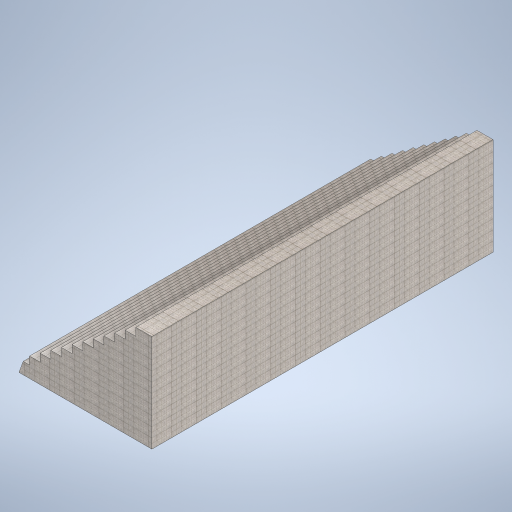
# Autodesk Inventor part: front_stair
Saved by Autodesk Inventor 2024.2 (Build 282272000, 272)
## iProperties
Created: 2024-05-25
Part Number: front_stair
Material: Generic
Document SubType Name: Modeling
Designer: LOSTER_1
Density: 1 g/cm^3
Appearance: Default
Author: LOSTER_1
Autodesk Inventor part; units mm, degrees
ref_plane "YZ Plane" through (0, 0, 0) normal (1, 0, 0) x (0, 1, 0)
ref_plane "XZ Plane" through (0, 0, 0) normal (0, 1, 0) x (-1, 0, 0)
ref_plane "XY Plane" through (0, 0, 0) normal (0, 0, 1) x (1, 0, 0)
sketch "Sketch1" plane through (0, 0, 0) normal (0, 1, 0) x (-1, 0, 0)
  line L0 (1000, 3500) -> (-1000, 3500)
  line L1 (-1000, 3500) -> (-1000, -3500)
  line L2 (-1000, -3500) -> (1000, -3500)
  line L3 (1000, -3500) -> (1000, 3500)
  line L4 (1000, 3500) -> (-1000, -3500) construction
  line L5 (-1000, 3500) -> (1000, -3500) construction
  point P0 (0, 0)
  dimension "d0" = 2000
  dimension "d1" = 7000
  constraints: 12 end point, 2 midpoint, 2 parallel, 1 horizontal, 1 perpendicular
  measures "d0" distance of L2.end L1.end
  measures "d1" distance of L1.end L0.end
extrude "Extrusion1" add sketch "Sketch1" along normal blind 2000
sketch "Sketch2" plane through (-1000, 0, 3500) normal (0, 0, 1) x (1, 0, 0)
  line L0 (2000, 2000) -> (0, 2000) projected
  line L1 (0, 2000) -> (0, 0)
  line L2 (0, 0) -> (-727.9405, 0)
  line L3 (2000, 0) -> (0, 0) projected
  line L4 (0, 2000) -> (-727.9405, 0)
  line L5 (0, 2000) -> (2128.3555, 2000) construction
  point P0 (1000, 0)
  dimension "d4" = 110
  constraints: 8 end point, 1 collinear, 1 equal length, 1 horizontal, 1 vertical
  measures "d4" angle of L4 L5
extrude "Extrusion2" add sketch "Sketch2" against normal blind 7000
sketch "Sketch3" plane through (1000, 0, 3500) normal (0, 0, 1) x (1, 0, 0)
  line L0 (0, 0) -> (0, 2000) projected
  line L1 (0, 0) -> (0, 160)
  line L2 (0, 160) -> (0, 320)
  line L3 (0, 320) -> (0, 480)
  line L4 (0, 480) -> (0, 640)
  line L5 (0, 640) -> (0, 800)
  line L6 (0, 800) -> (0, 960)
  line L7 (0, 960) -> (0, 1120)
  line L8 (0, 1120) -> (0, 1280)
  line L9 (0, 1280) -> (0, 1440)
  line L10 (0, 1440) -> (0, 1600)
  line L11 (0, 1600) -> (0, 1760)
  line L12 (0, 1760) -> (0, 1920)
  line L13 (0, 1920) -> (0, 2000.3283)
  line L14 (0, 0) -> (-2727.9405, 0) projected
  line L15 (-2727.9405, 0) -> (-2509.9405, 0)
  line L16 (-2509.9405, 0) -> (-2291.9405, 0)
  line L17 (-2291.9405, 0) -> (-2073.9405, 0)
  line L18 (-2073.9405, 0) -> (-1855.9405, 0)
  line L19 (-1855.9405, 0) -> (-1637.9405, 0)
  line L20 (-1637.9405, 0) -> (-1419.9405, 0)
  line L21 (-1419.9405, 0) -> (-1201.9405, 0)
  line L22 (-1201.9405, 0) -> (-983.9405, 0)
  line L23 (-983.9405, 0) -> (-765.9405, 0)
  line L24 (-765.9405, 0) -> (-547.9405, 0)
  line L25 (-547.9405, 0) -> (-329.9405, 0)
  line L26 (-329.9405, 0) -> (-111.9405, 0)
  line L27 (-111.9405, 0) -> (0, 0)
  line L28 (-2727.9405, 0) -> (-2640.5876, 240)
  line L29 (-2727.9405, 0) -> (-2000, 2000) projected
  line L30 (-2640.5876, 240) -> (-2509.9405, 240)
  line L31 (-2509.9405, 240) -> (-2509.9405, 400)
  line L32 (-2509.9405, 400) -> (-2291.9405, 400)
  line L33 (-2291.9405, 400) -> (-2291.9405, 560)
  line L34 (-2291.9405, 560) -> (-2073.9405, 560)
  line L35 (-2073.9405, 560) -> (-2073.9405, 720)
  line L36 (-2073.9405, 720) -> (-1855.9405, 720)
  line L37 (-1855.9405, 720) -> (-1855.9405, 880)
  line L38 (-1855.9405, 880) -> (-1637.9405, 880)
  line L39 (-1637.9405, 880) -> (-1637.9405, 1040)
  line L40 (-1637.9405, 1040) -> (-1419.9405, 1040)
  line L41 (-1419.9405, 1040) -> (-1419.9405, 1200)
  line L42 (-1419.9405, 1200) -> (-1201.9405, 1200)
  line L43 (-1201.9405, 1200) -> (-1201.9405, 1360)
  line L44 (-1201.9405, 1360) -> (-983.9405, 1360)
  line L45 (-983.9405, 1360) -> (-983.9405, 1520)
  line L46 (-983.9405, 1520) -> (-765.9405, 1520)
  line L47 (-765.9405, 1520) -> (-765.9405, 1680)
  line L48 (-765.9405, 1680) -> (-547.9405, 1680)
  line L49 (-547.9405, 1680) -> (-547.9405, 1840)
  line L50 (-547.9405, 1840) -> (-329.9405, 1840)
  line L51 (-329.9405, 1840) -> (-329.9405, 2000)
  line L52 (-329.9405, 2000) -> (-2000, 2000)
  line L53 (-2000, 2000) -> (-2640.5876, 240)
  point P0 (-1000, 0)
  dimension "d7" = 160
  dimension "d8" = 160
  dimension "d9" = 160
  dimension "d10" = 160
  dimension "d11" = 160
  dimension "d12" = 160
  dimension "d13" = 160
  dimension "d14" = 160
  dimension "d15" = 160
  dimension "d16" = 160
  dimension "d17" = 160
  dimension "d18" = 160
  dimension "d19" = 218
  dimension "d20" = 218
  dimension "d21" = 218
  dimension "d22" = 218
  dimension "d23" = 218
  dimension "d24" = 218
  dimension "d25" = 218
  dimension "d26" = 218
  dimension "d27" = 218
  dimension "d28" = 218
  dimension "d29" = 218
  dimension "d30" = 218
  constraints: 102 end point, 22 perpendicular, 13 coincident, 4 point on line, 2 horizontal, 1 collinear, 24 other
  measures "d7" distance of L1.start L1.end
  measures "d8" distance of L1.end L2.end
  measures "d9" distance of L2.end L3.end
  measures "d10" distance of L3.end L4.end
  measures "d11" distance of L4.end L5.end
  measures "d12" distance of L5.end L6.end
  measures "d13" distance of L6.end L7.end
  measures "d14" distance of L7.end L8.end
  measures "d15" distance of L8.end L9.end
  measures "d16" distance of L9.end L10.end
  measures "d17" distance of L10.end L11.end
  measures "d18" distance of L11.end L12.end
  measures "d19" distance of L15.start L15.end
  measures "d20" distance of L15.end L16.end
  measures "d21" distance of L16.end L17.end
  measures "d22" distance of L17.end L18.end
  measures "d23" distance of L18.end L19.end
  measures "d24" distance of L19.end L20.end
  measures "d25" distance of L20.end L21.end
  measures "d26" distance of L21.end L22.end
  measures "d27" distance of L22.end L23.end
  measures "d28" distance of L23.end L24.end
  measures "d29" distance of L24.end L25.end
  measures "d30" distance of L25.end L26.end
extrude "Extrusion3" cut sketch "Sketch3" against normal through all
body "Solid1"
